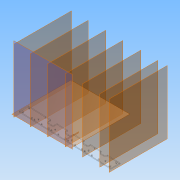
# Autodesk Inventor part: Pancake_Reverse Backboard
Saved by Autodesk Inventor 2018.1 (Build 221171000, 171)
## iProperties
Created: 2019-02-22
Part Number: Pancake_Reverse Backboard
Material: PET Plastic
Document SubType Name: Modeling
Designer: James
Density: 1.541 g/cm^3
Appearance: Polycarbonate - Clear
Author: James
Autodesk Inventor part; units mm, degrees
ref_plane "YZ Plane" through (0, 0, 0) normal (1, 0, 0) x (0, 1, 0)
ref_plane "XZ Plane" through (0, 0, 0) normal (0, 1, 0) x (-1, 0, 0)
ref_plane "XY Plane" through (0, 0, 0) normal (0, 0, 1) x (1, 0, 0)
derived "Pancake_Skeleton.ipt"
ref_plane "Ground" through (0, 0, 0) normal (0, 1, 0) x (-1, 0, 0)
ref_plane "Back" through (0, 0, 0) normal (0, 0, 1) x (1, 0, 0)
ref_plane "LHS" through (0, 0, 0) normal (1, 0, 0) x (0, 1, 0)
ref_plane "Lane 1" through (90, 0, 0) normal (1, 0, 0) x (0, 1, 0)
ref_plane "Lane 2" through (185, 0, 0) normal (1, 0, 0) x (0, 1, 0)
ref_plane "Lane 3" through (280, 0, 0) normal (1, 0, 0) x (0, 1, 0)
ref_plane "Lane 4" through (375, 0, 0) normal (1, 0, 0) x (0, 1, 0)
ref_plane "Lane 5" through (470, 0, 0) normal (1, 0, 0) x (0, 1, 0)
ref_plane "RHS" through (520, 0, 0) normal (1, 0, 0) x (0, 1, 0)
sketch "Sketch1" plane through (0, 0, 0) normal (0, 0, 1) x (1, 0, 0)
  line L0 (0, 84) -> (0, -14) projected
  line L1 (520, 84) -> (520, -14) projected
  line L2 (0, 20) -> (520, 0)
  line L3 (520, 0) -> (520, 50)
  line L4 (520, 50) -> (0, 70)
  line L5 (0, 70) -> (0, 20)
  line L6 (-104, 0) -> (624, 0) projected
  dimension "d31" = 50
  dimension "d32" = 20
  constraints: 8 end point, 2 parallel, 2 point on line, 1 collinear, 1 vertical
  measures "d31" distance of L2.end L3.end
  measures "d32" vertical distance of L2.end L2.start
extrude "Extrusion1" add sketch "Sketch1" along normal blind 5 contours L4 L1 L2 L0
sketch "Sketch2" plane through (0, 0, 5) normal (0, 0, 1) x (1, 0, 0)
  line L0 (90, 84) -> (90, -14) projected
  line L1 (520, 50) -> (0, 70) projected
  line L2 (-104, 0) -> (624, 0) projected
  line L3 (185, 84) -> (185, -14) projected
  line L4 (0, 84) -> (0, -14) projected
  line L5 (0, 20) -> (520, 0) projected
  point P0 (0, 0)
  point P1 (50, 58.0769)
  point P2 (50, 28.0769)
  dimension "d4" = 30
  dimension "d29" = 95
  dimension "d30" = 50
  dimension "d33" = 9.9926
  dimension "d34" = 9.9926
  constraints: 1 vertical alignment
  measures "d4" distance of point (50, 28.077) point (50, 58.077)
  measures "d29" distance between parallel lines of L3 L0
  measures "d30" distance from line of point (50, 58.077) L4
  measures "d33" distance from line of L1 point (50, 58.077)
  measures "d34" distance from line of L5 point (50, 28.077)
hole "Hole1" [suppressed]
pattern_linear "Rectangular Pattern1" [suppressed]
sketch "Sketch3" plane through (0, 0, 5) normal (0, 0, 1) x (1, 0, 0)
  line L0 (520, 50) -> (0, 70) projected
  line L1 (-104, 0) -> (624, 0) projected
  line L2 (0, 84) -> (0, -14) projected
  line L3 (0, 20) -> (520, 0) projected
  line L4 (520, 84) -> (520, -14) projected
  point P0 (0, 0)
  point P1 (12.5, 62.5)
  point P2 (12.5, 27.5)
  point P3 (507.5, 42.5)
  point P4 (507.5, 7.5)
  dimension "d20" = 12.5
  dimension "d36" = 35
  dimension "d38" = 12.5
  dimension "d39" = 35
  dimension "d41" = 7.5
  dimension "d42" = 7.5
  constraints: 2 vertical alignment
  measures "d20" distance from line of L2 point (12.5, 62.5)
  measures "d36" distance of point (12.5, 27.5) point (12.5, 62.5)
  measures "d38" distance from line of L4 point (507.5, 42.5)
  measures "d39" distance of point (507.5, 7.5) point (507.5, 42.5)
  measures "d41" vertical distance of L0.start point (507.5, 42.5)
  measures "d42" vertical distance of point (12.5, 62.5) L0.end
hole "Hole2" at (12.5, 62.5, 5) at (12.5, 27.5, 5) at (507.5, 42.5, 5) at (507.5, 7.5, 5) direction (0, 0, -1) diameter 4.5 end through all countersink diameter 9.4 countersink angle 90 clearance for "Flat Head Machine Screw" size "M4" standard "Ansi Metric M Profile"
ref_plane "Work Plane10" through (260, 20, 0) normal (-1, 0, 0) x (0, 0, 1)
sketch "Sketch4" plane through (0, 0, 5) normal (0, 0, 1) x (1, 0, 0)
  line L0 (80, 59.4175) -> (78.6548, 24.4434)
  line L1 (479.7045, 44.0443) -> (478.3593, 9.0701)
  line L2 (520, 50) -> (0, 70) projected
  line L3 (0, 20) -> (520, 0) projected
  line L4 (0, 84) -> (0, -14) projected
  line L5 (520, 84) -> (520, -14) projected
  point P0 (0, 0)
  dimension "d43" = 7.5
  dimension "d44" = 7.5
  dimension "d48" = 35
  dimension "d49" = 80
  dimension "d58" = 35
  dimension "d60" = 400
  constraints: 4 end point, 2 perpendicular
  measures "d43" distance from line of L2 L0.start
  measures "d44" distance from line of L2 L1.start
  measures "d48" distance of L0.start L0.end
  measures "d49" distance from line of L0.start L4
  measures "d58" distance of L1.start L1.end
  measures "d60" distance of L1.start L0.start
hole "Hole3" [suppressed]
sketch "Sketch5" plane through (0, 0, 5) normal (0, 0, 1) x (1, 0, 0)
  line L0 (0, 84) -> (0, -14) projected
  line L1 (520, 84) -> (520, -14) projected
  line L2 (520, 50) -> (0, 70) projected
  point P0 (0, 0)
  point P1 (100, 62.1509)
  point P2 (379.7931, 51.3896)
  dimension "d61" = 280
  dimension "d62" = 100
  dimension "d64" = 4
  dimension "d65" = 4
  dimension "d66" = 140.2069
  measures "d61" distance of point (379.793, 51.39) point (100, 62.151)
  measures "d62" distance from line of L0 point (100, 62.151)
  measures "d64" distance from line of L2 point (379.793, 51.39)
  measures "d65" distance from line of point (100, 62.151) L2
  measures "d66" distance from line of L1 point (379.793, 51.39)
hole "Hole4" at (100, 62.1509, 5) at (379.7931, 51.3896, 5) direction (0, 0, -1) diameter 3.4 end through all clearance for "Flat Head Machine Screw" size "M3" standard "Ansi Metric M Profile"
sketch "Sketch6" plane through (0, 0, 5) normal (0, 0, 1) x (1, 0, 0)
  line L0 (0, 20) -> (520, 0) projected
  line L1 (90, 84) -> (90, -14) projected
  point P0 (0, 0)
  point P1 (65, 24.0048)
  dimension "d74" = 6.5
  dimension "d75" = 25
  measures "d74" distance from line of L0 point (65, 24.005)
  measures "d75" distance from line of L1 point (65, 24.005)
hole "Hole5" at (65, 24.0048, 5) direction (0, 0, -1) diameter 7 end through all
pattern_linear "Rectangular Pattern2" count 5 spacing 95 along (0.9992612, -0.0384331, 0) of "Hole5"
sketch "Sketch7" plane through (0, 0, 5) normal (0, 0, 1) x (1, 0, 0)
  circle A0 centre (47, 14.0048) radius 12.5
  circle A1 centre (65, 24.0048) radius 3.5 projected
  point P0 (0, 0)
  dimension "d86" = 18
  dimension "d87" = 10
  dimension "d88" = 25
  constraints: 1 centre point
  measures "d86" horizontal distance of A1.centre A0.centre
  measures "d87" vertical distance of A1.centre A0.centre
  measures "d88" diameter of A0
extrude "Extrusion2" [suppressed]
pattern_linear "Rectangular Pattern3" [suppressed]
sketch "Sketch8" plane through (0, 0, 5) normal (0, 0, 1) x (1, 0, 0)
  line L0 (127.5, 72.5) -> (162.5, 72.5)
  line L1 (162.5, 72.5) -> (162.5, 42.5)
  line L2 (162.5, 42.5) -> (127.5, 42.5)
  line L3 (127.5, 42.5) -> (127.5, 72.5)
  line L4 (0, 87) -> (0, -14.5) projected
  circle A0 centre (12.5, 62.5) radius 2.25 projected
  line L5 (90, 87) -> (90, -14.5) projected
  point P0 (0, 0)
  dimension "d94" = 35
  dimension "d104" = 10
  dimension "d105" = 30
  dimension "d132" = 37.5
  constraints: 8 end point, 2 parallel, 1 horizontal, 1 perpendicular
  measures "d94" distance of L0.start L0.end
  measures "d104" distance from line of A0.centre L0
  measures "d105" distance between parallel lines of L0 L2
  measures "d132" distance between parallel lines of L3 L5
extrude "Extrusion3" cut sketch "Sketch8" against normal through all contours L0 L1 L2 L3
fillet "Fillet1" radius 10 2 edges at (162.5, 42.5, 2.5) (127.5, 42.5, 2.5)
pattern_linear "Rectangular Pattern4" count 4 spacing 95 along (1, 0, 0) of "Extrusion3", "Fillet1"
sketch "Sketch9" plane through (0, 0, 5) normal (0, 0, 1) x (1, 0, 0)
  circle A0 centre (65, 24.0048) radius 3.5 projected
  point P0 (0, 0)
  point P1 (90, 35.0048)
  dimension "d106" = 11
  dimension "d107" = 25
  measures "d106" vertical distance of point (90, 35.005) A0.centre
  measures "d107" horizontal distance of point (90, 35.005) A0.centre
hole "Hole6" at (90, 35.0048, 5) direction (0, 0, -1) diameter 3.4 end through all countersink diameter 6.3 countersink angle 90 clearance for "Flat Head Machine Screw" size "M3" standard "Ansi Metric M Profile"
pattern_linear "Rectangular Pattern5" count 5 spacing 95 along (0.9992612, -0.0384331, 0) of "Hole6"
sketch "Sketch10" plane through (0, 0, 0) normal (0, 0, -1) x (-1, 0, 0)
  line L0 (0, 20) -> (-520, 0) projected
  circle A0 centre (-65, 24.0048) radius 3.5 projected
  point P0 (0, 0)
  point P1 (-80, 23.9283)
  point P2 (-119.9704, 22.3909)
  dimension "d118" = 7
  dimension "d119" = 7
  dimension "d120" = 15
  dimension "d121" = 40
  measures "d118" distance from line of L0 point (-80, 23.928)
  measures "d119" distance from line of L0 point (-119.97, 22.391)
  measures "d120" horizontal distance of point (-80, 23.928) A0.centre
  measures "d121" distance of point (-119.97, 22.391) point (-80, 23.928)
hole "Hole7" at (80, 23.9283, 0) at (119.9704, 22.3909, 0) direction (0, 0, 1) diameter 3.4 end through all countersink diameter 6.3 countersink angle 90 clearance for "Flat Head Machine Screw" size "M3" standard "Ansi Metric M Profile"
pattern_linear "Rectangular Pattern6" count 4 spacing 95 along (0.9992612, -0.0384331, 0) of "Hole7"
equation "\"d33\" = d34"
equation "\"d44\" = d43"
equation "\"d58\" = d48"
equation "\"d65\" = d64"
equation "\"d119\" = d118"
body "Solid1"
